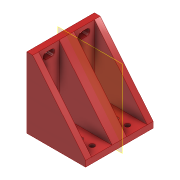
# Autodesk Inventor part: Cross bar bracket generic
Saved by Autodesk Inventor 2020 (Build 240168000, 168)
## iProperties
Created: 2019-12-28
Part Number: Cross bar bracket generic
Material: Generic
Document SubType Name: Modeling
Designer: ball
Density: 1 g/cm^3
Appearance: Default
Author: ball
Autodesk Inventor part; units mm, degrees
ref_plane "YZ Plane" through (0, 0, 0) normal (1, 0, 0) x (0, 1, 0)
ref_plane "XZ Plane" through (0, 0, 0) normal (0, 1, 0) x (-1, 0, 0)
sketch "Sketch1" plane through (0, 0, 0) normal (0, 1, 0) x (-1, 0, 0)
  line L0 (-40, -23) -> (0, -23)
  line L1 (-40, 23) -> (0, 23)
  line L2 (0, 23) -> (0, -23)
  line L3 (-40, 23) -> (-40, -23)
  line L4 (-40, -12) -> (0, -12) construction
  line L5 (-40, 12) -> (0, 12) construction
  circle A0 centre (-9.5, 12) radius 1.7
  line L6 (-4, 23) -> (-4, -23) construction
  circle A1 centre (-17.5, 12) radius 1.7
  circle A2 centre (-25.5, 12) radius 1.7
  circle A3 centre (-33.5, 12) radius 1.7
  circle A4 centre (-9.5, -12) radius 1.7
  circle A5 centre (-17.5, -12) radius 1.7
  circle A6 centre (-25.5, -12) radius 1.7
  circle A7 centre (-33.5, -12) radius 1.7
  circle A8 centre (-9.5, 12) radius 3.5 construction
  line L7 (0, 19) -> (-40, 19) construction
  point P0 (0, 0)
  dimension "d5" = 46
  dimension "d6" = 23
  dimension "d7" = 40
  dimension "d8" = 0
  dimension "d9" = 12
  dimension "d10" = 12
  dimension "d11" = 3.4
  dimension "d12" = 4
  dimension "d13" = 9.5
  dimension "d16" = 8
  dimension "d19" = 24
  dimension "d22" = 7
  dimension "d23" = 4
  constraints: 16 end point, 9 centre point, 7 point on line, 3 perpendicular, 2 vertical, 1 coincident, 1 horizontal, 1 parallel, 14 other
  measures "d5" distance between parallel lines of L0 L1
  measures "d6" distance from line of L0 point (0, 0)
  measures "d7" distance between parallel lines of L3 L2
  measures "d8" distance from line of L2 point (0, 0)
  measures "d9" distance from line of L5 point (0, 0)
  measures "d10" distance from line of L4 point (0, 0)
  measures "d11" diameter of A0
  measures "d12" distance between parallel lines of L6 L2
  measures "d13" distance from line of L2 A0.centre
  measures "d16" distance of A0.centre A1.centre
  measures "d19" distance of A0.centre A4.centre
  measures "d22" diameter of A8
  measures "d23" distance between parallel lines of L7 L1
extrude "Lift Attachment Plate" add sketch "Sketch1" along normal blind 4
sketch "Sketch2" plane through (0, 4, 0) normal (0, 1, 0) x (1, 0, 0)
  line L0 (0, 23) -> (0, -23) projected
  line L1 (40, 23) -> (0, 23) projected
  line L2 (0, -23) -> (4, -23)
  line L3 (4, -23) -> (4, 23)
  line L4 (4, 23) -> (0, 23)
  line L5 (0, 23) -> (0, -23)
  point P0 (0, 0)
  dimension "d26" = 4
  constraints: 8 end point, 2 parallel, 1 horizontal, 1 perpendicular, 1 point on line
  measures "d26" distance of L4.end L3.end
extrude "Cross bar Attachment Plate" add sketch "Sketch2" along normal blind 44
sketch "Sketch3" plane through (0, 0, 23) normal (0, 0, 1) x (1, 0, 0)
  line L0 (4, 4) -> (4, 48) projected
  line L1 (4, 48) -> (4, 4)
  line L2 (40, 4) -> (4, 4) projected
  line L3 (4, 4) -> (40, 4)
  line L4 (40, 4) -> (4, 48)
  point P0 (0, 0)
  constraints: 6 end point, 2 collinear
extrude "Left bracket" add sketch "Sketch3" against normal blind 4
sketch "Sketch4" plane through (0, 0, 0) normal (0, 0, 1) x (1, 0, 0)
  line L0 (4, 48) -> (40, 4) projected
  line L1 (4, 4) -> (40, 4) projected
  line L2 (4, 48) -> (4, 4)
  line L3 (4, 4) -> (40, 4)
  line L4 (40, 4) -> (4, 48)
  point P0 (0, 0)
  constraints: 6 end point, 1 collinear, 1 vertical
extrude "Center bracket" add sketch "Sketch4" along normal mid plane 10
sketch "Sketch5" plane through (40, 0, -23) normal (0, 0, -1) x (-1, 0, 0)
  line L0 (36, 48) -> (40, 48) projected
  line L1 (36, 48) -> (36, 4) projected
  line L2 (36, 48) -> (36, 4)
  line L3 (0, 4) -> (36, 4) projected
  line L4 (36, 4) -> (0, 4)
  line L5 (0, 4) -> (36, 48)
  point P0 (40, 0)
  constraints: 6 end point, 1 collinear, 1 vertical
extrude "Right bracket" add sketch "Sketch5" against normal blind 4
sketch "Sketch6" plane through (0, 0, -23) normal (-1, 0, 0) x (0, 0, 1)
  circle A0 centre (35, 11) radius 2 construction
  circle A1 centre (11, 11) radius 2 construction
  line L0 (0, 0) -> (46, 0) construction
  line L1 (23, 57.6) -> (23, -9.6) construction
  circle A2 centre (35, 43) radius 2 construction
  circle A3 centre (11, 43) radius 2 construction
  line L2 (42, 48) -> (42, 4) construction
  line L3 (4, 4) -> (4, 48) construction
  line L4 (15, 11) -> (7, 11) construction
  line L5 (4, 4) -> (4, 48) projected
  line L6 (12.8, 13.2) -> (9.2, 13.2)
  line L7 (9.2, 8.8) -> (12.8, 8.8)
  arc A4 (12.8, 8.8) -> (12.8, 13.2) centre (12.8, 11) ccw
  arc A5 (9.2, 13.2) -> (9.2, 8.8) centre (9.2, 11) ccw
  point P0 (23, 0)
  dimension "d35" = 4
  dimension "d36" = 4
  dimension "d37" = 11
  dimension "d38" = 11
  dimension "d39" = 12
  dimension "d40" = 12
  dimension "d41" = 4
  dimension "d42" = 4
  dimension "d43" = 32
  dimension "d44" = 32
  dimension "d45" = 4
  dimension "d46" = 4
  dimension "d47" = 4.4
  constraints: 8 end point, 6 centre point, 6 point on circle, 4 tangent, 2 point on line, 1 horizontal, 1 midpoint, 1 parallel, 1 other
  measures "d35" diameter of A0
  measures "d36" diameter of A1
  measures "d37" distance from line of L0 A0.centre
  measures "d38" distance from line of L0 A1.centre
  measures "d39" distance from line of L1 A1.centre
  measures "d40" distance from line of L1 A0.centre
  measures "d41" diameter of A2
  measures "d42" diameter of A3
  measures "d43" distance of A0.centre A2.centre
  measures "d44" distance of A3.centre A1.centre
  measures "d45" distance of A1.centre L4.end
  measures "d46" distance of A1.centre L4.start
  measures "d47" diameter of A5
extrude "Extrusion6" cut sketch "Sketch6" against normal through all
pattern_linear "Rectangular Pattern1" count 2 spacing 24 along (0, 0, 1) count 2 spacing 32 along (0, 1, 0) of "Extrusion6"
equation "\"d6\" = 0.5 * d5"
equation "\"d10\" = d9"
equation "\"d38\" = d37"
equation "\"d39\" = d40"
equation "\"d44\" = d43"
equation "\"d46\" = d45"
body "Solid1"
